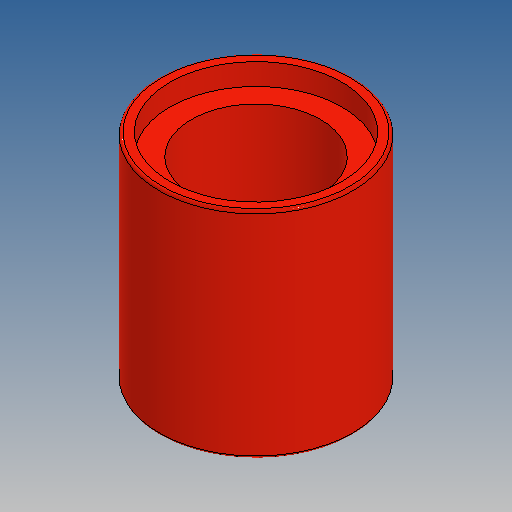
# Autodesk Inventor part: 18654-Red
Saved by Autodesk Inventor 2025 (Build 290162010, 162A)
## iProperties
Created: 2015-02-02
Part Number: 18654-Red
Material: ABS Plastic
Document SubType Name: Modeling
Designer: D. Kohfeld
Mass: 0.171197 g
Surface Area: 3.51918 cm^2
Volume: 0.161507 cm^3
Density: 1.06 g/cm^3
Appearance: Red
Author: D. Kohfeld
Autodesk Inventor part; units mm, degrees
ref_plane "YZ Plane" through (0, 0, 0) normal (1, 0, 0) x (0, 1, 0)
ref_plane "XZ Plane" through (0, 0, 0) normal (0, 1, 0) x (-1, 0, 0)
ref_plane "XY Plane" through (0, 0, 0) normal (0, 0, 1) x (1, 0, 0)
sketch "Sketch1" plane through (0, 0, 0) normal (0, 0, 1) x (1, 0, 0)
  line L0 (0, -5.6) -> (0, 5.6) projected
  line L1 (2.4, -3.2) -> (2.4, 3.2)
  line L2 (2.4, 3.2) -> (3.2, 3.2)
  line L3 (3.2, 3.2) -> (3.2, 4)
  line L4 (3.2, 4) -> (3.6, 4)
  line L5 (3.6, 4) -> (3.6, -4)
  line L6 (3.6, -4) -> (3.2, -4)
  line L7 (3.2, -4) -> (3.2, -3.2)
  line L8 (3.2, -3.2) -> (2.4, -3.2)
  point P0 (0, 0)
  point P1 (2.4, 0)
  dimension "d0" = 4.8
  dimension "d1" = 8
  dimension "d2" = 6.4
  dimension "d3" = 0.8
  dimension "d4" = 7.2
  constraints: 16 end point, 7 parallel, 2 equal length, 1 horizontal alignment, 1 midpoint, 1 perpendicular
  measures "d0" diameter of L1 L0
  measures "d1" distance of L4.end L5.end
  measures "d2" diameter of L3 L0
  measures "d3" distance between parallel lines of L2 L4
  measures "d4" diameter of L5 L0
revolve "Revolution1" add sketch "Sketch1" angle 360 about axis through (0, -10, 0) along (0, 1, 0)
fillet "Fillet1" radius 0.1 2 edges at (-3.6, 4, 0) (-3.6, -4, 0)
equation "\"d0\" = tpd"
equation "\"d1\" = lu"
equation "\"d2\" = tsd"
equation "\"d3\" = tsl"
equation "\"d4\" = tlad"
equation "\"tpd\" = 4.8"
equation "\"lu\" = 8"
equation "\"tsd\" = 6.4"
equation "\"tsl\" = 0.8"
equation "\"tlad\" = 7.2"
body "Solid1"
